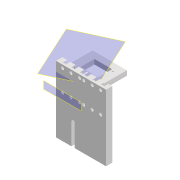
# Autodesk Inventor part: 30_cellSTORM_UC2_Laser_holder
Saved by Autodesk Inventor 2022 (Build 260153000, 153)
## iProperties
Created: 2021-11-15
Part Number: 30_cellSTORM_UC2_Laser_holder
Material: Generic
Document SubType Name: Modeling
Designer: diederichbenedict
Density: 1 g/cm^3
Appearance: Default
Author: diederichbenedict
Autodesk Inventor part; units mm, degrees
ref_plane "YZ Plane" through (0, 0, 0) normal (1, 0, 0) x (0, 1, 0)
ref_plane "XZ Plane" through (0, 0, 0) normal (0, 1, 0) x (-1, 0, 0)
ref_plane "Work Plane1" through (22.2, 37.1, 6) normal (0, 0, -1) x (0, 1, 0)
ref_plane "Work Plane2" through (0, 0, 0) normal (0, 0, 1) x (1, 0, 0)
sketch "Sketch1" plane through (22.2, 37.1, 6) normal (0, 0, -1) x (0, 1, 0)
  circle A0 centre (25.9, 3.8) radius 1.75
  circle A1 centre (25.9, -16.2) radius 1.75
  circle A2 centre (5.9, 3.8) radius 1.75
  circle A3 centre (5.9, -16.2) radius 1.5
  line L0 (3, -22.4) -> (9.5, -22.4) construction
  line L1 (9.5, 10) -> (9.5, -22.4) construction
  line L2 (3, 10) -> (9.5, 10) construction
  line L3 (3, 10) -> (3, -22.4) construction
  circle A4 centre (5.9, 3.8) radius 1.75 construction
  circle A5 centre (5.9, -16.2) radius 1.75 construction
  line L4 (28.8, -22.4) -> (21.9, -22.4) construction
  line L5 (21.9, 10) -> (21.9, -22.4) construction
  line L6 (28.8, 10) -> (21.9, 10) construction
  line L7 (28.8, 10) -> (28.8, -22.4) construction
  line L8 (19.9, 3.8) -> (19.9, -14.6723) construction
  line L9 (28.8, 10) -> (-33.8945, 10)
  line L10 (-33.8945, 10) -> (-33.8945, -22.4)
  line L11 (-33.8945, -22.4) -> (28.8, -22.4)
  line L12 (28.8, -22.4) -> (28.8, 10)
  line L13 (-33.8945, -22.4) -> (28.8, -22.4)
  line L14 (28.8, -22.4) -> (28.8, -37.4)
  line L15 (28.8, -37.4) -> (-33.8945, -37.4)
  line L16 (-33.8945, -37.4) -> (-33.8945, -22.4)
  line L17 (28.8, 10) -> (-33.8945, 10)
  line L18 (-33.8945, 10) -> (-33.8945, 25)
  line L19 (-33.8945, 25) -> (28.8, 25)
  line L20 (28.8, 25) -> (28.8, 10)
  line L21 (28.8, 25) -> (-33.8945, 10)
  point P0 (-37.1, -22.2)
  point P1 (28.8, -22.4)
extrude "Extrusion1" add sketch "Sketch1" along normal up to surface (6 mm away) contours A0 | A1 | A2 | A3 | L12 L11 L10 L9 | L9 L21 L20 | L18 L19 L21
sketch "Sketch2" plane through (22.2, 37.1, 6) normal (0, 0, 1) x (1, 0, 0)
  line L0 (10, 28.8) -> (10, -33.8945) projected
  circle A0 centre (-6.2, -29.1) radius 1.4 projected
  line L1 (-6.2, -54.7229) -> (-6.2, -13.0662) construction
  line L2 (10, -33.8945) -> (-22.4, -33.8945) projected
  line L3 (-4.7, -54.7229) -> (-4.7, -13.0662)
  line L4 (-7.7, -13.0662) -> (-7.7, -54.7229)
  arc A1 (-7.7, -54.7229) -> (-4.7, -54.7229) centre (-6.2, -54.7229) ccw
  arc A2 (-4.7, -13.0662) -> (-7.7, -13.0662) centre (-6.2, -13.0662) ccw
  line L5 (10, -33.8945) -> (-37.4, -33.8945) projected
  line L6 (-37.4, 28.8) -> (10, 28.8) projected
  line L7 (-37.4, -33.8945) -> (-37.4, 28.8) projected
  point P0 (-22.2, -37.1)
  point P1 (-6.2, -33.8945)
  dimension "d2" = 3
  constraints: 8 end point, 4 point on circle, 4 tangent, 2 centre point, 2 midpoint, 1 parallel, 1 perpendicular
  measures "d2" diameter of A2
extrude "Extrusion2" cut sketch "Sketch2" against normal blind 10 contours L3 A1 L4 L2 | L2 L4 A2 L3 | A0
sketch "Sketch3" plane through (32.2, 65.9, 0) normal (0, 0, -1) x (-1, 0, 0)
  circle A0 centre (6.2, -22.9) radius 1.25 projected
  circle A1 centre (26.2, -22.9) radius 1.25 projected
  circle A2 centre (26.2, -2.9) radius 1.25 projected
  circle A3 centre (6.2, -2.9) radius 1.25 projected
  line L0 (47.4, 0) -> (0, 0) projected
  point P0 (32.2, -65.9)
  point P1 (14.2, -22.9)
  point P2 (34.2, -22.9)
  point P3 (34.2, -2.9)
  point P4 (14.2, -2.9)
  point P5 (22.2, -22.9)
  point P6 (42.2, -22.9)
  point P7 (42.2, -2.9)
  point P8 (22.2, -2.9)
  dimension "d22" = 8
  constraints: 1 horizontal, 8 other
  measures "d22" distance of A0.centre point (14.2, -22.9)
hole "Hole1" at (6, 63, 0) at (26, 63, 0) at (26, 43, 0) at (6, 43, 0) at (-10, 43, 0) at (-2, 43, 0) at (-2, 63, 0) at (-10, 63, 0) direction (0, 0, 1) diameter 2.9 end through all counterbore diameter 6.5 counterbore depth 4
ref_plane "Work Plane3" through (0.2759, 57, -15.7452) normal (0, -1, 0) x (-0.9087, 0, 0.4175)
sketch "Sketch4" plane through (32.2, 3.2055, 0) normal (0, 0, -1) x (-1, 0, 0)
  line L0 (41.88, 53.7945) -> (-24.48, 53.7945) projected
  line L1 (32.4, 0) -> (32.4, 37.0885) projected
  line L2 (0, 62.6945) -> (0, 0) projected
  line L3 (32.4, 53.7945) -> (0, 53.7945)
  line L4 (0, 53.7945) -> (0, 49.2945)
  line L5 (0, 49.2945) -> (32.4, 49.2945)
  line L6 (32.4, 49.2945) -> (32.4, 53.7945)
  line L7 (32.4, 62.6945) -> (-15, 62.6945) projected
  line L8 (32.4, 62.6945) -> (0, 62.6945)
  line L9 (0, 62.6945) -> (0, 57.6945)
  line L10 (0, 57.6945) -> (32.4, 57.6945)
  line L11 (32.4, 57.6945) -> (32.4, 62.6945)
  point P0 (32.2, -3.2055)
  point P1 (26.2, 47.7945)
  point P2 (32.4, 49.2945)
  point P3 (0, 53.7945)
  point P4 (0, 53.7945)
  dimension "d12" = 4.5
  dimension "d31" = 5
  constraints: 16 end point, 4 parallel, 4 point on line, 2 horizontal, 2 perpendicular, 1 other
  measures "d12" distance of L4.end L3.end
  measures "d31" distance of L9.end L8.end
pattern_linear "Rechteckige Anordnung1" count 3 spacing 8 along (1, 0, 0) of "Hole1"
extrude "Extrusion3" add sketch "Sketch4" along normal blind 28.7 and the other way blind 5 contours L2 L7 L11 L10
sketch "Sketch5" plane through (-0.2, 65.9, 0) normal (0, 1, 0) x (1, 0, 0)
  circle A0 centre (-1.3, 26) radius 1 projected
  circle A1 centre (26.7, 21) radius 1 construction
  circle A2 centre (5.2, 5.5) radius 1 construction
  circle A3 centre (16.2, 16) radius 2.6486 projected
  line L0 (24.5969, 9.4163) -> (7.8031, 9.4163)
  line L1 (7.8031, 9.4163) -> (7.8031, 22.5837)
  line L2 (7.8031, 22.5837) -> (24.5969, 22.5837)
  line L3 (24.5969, 22.5837) -> (24.5969, 9.4163)
  line L4 (24.5969, 9.4163) -> (7.8031, 22.5837) construction
  line L5 (7.8031, 9.4163) -> (24.5969, 22.5837) construction
  circle A4 centre (26.7, 21) radius 0.75
  circle A5 centre (5.2, 5.5) radius 0.75
  point P0 (0.2, 0)
  dimension "d15" = 1.5
  dimension "d16" = 1.5
  constraints: 12 end point, 2 centre point, 2 coincident, 2 midpoint, 2 parallel, 1 horizontal, 1 perpendicular
  measures "d15" diameter of A4
  measures "d16" diameter of A5
extrude "Extrusion4" cut sketch "Sketch5" against normal blind 10 contours A3 | L0 L1 L2 L3 | A4 | A5
body "Solid1"
